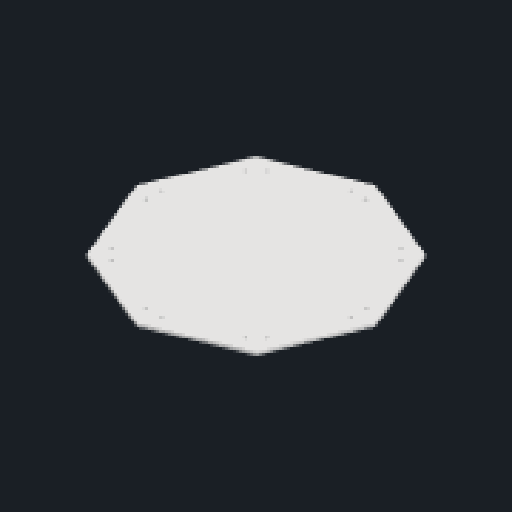
# Autodesk Inventor part: Bund
Saved by Autodesk Inventor 2026.2 (Build 302298000, 298)
## iProperties
Created: 2026-04-22
Part Number: Bund
Material: Generic
Document SubType Name: Modeling
Designer: Mikke
Density: 1 g/cm^3
Appearance: Default
Author: Mikke
Autodesk Inventor part; units mm, degrees
ref_plane "YZ Plane" through (0, 0, 0) normal (1, 0, 0) x (0, 1, 0)
ref_plane "XZ Plane" through (0, 0, 0) normal (0, 1, 0) x (-1, 0, 0)
ref_plane "XY Plane" through (0, 0, 0) normal (0, 0, 1) x (1, 0, 0)
sketch "Sketch1" plane through (0, 0, 0) normal (0, 1, 0) x (-1, 0, 0)
  line L0 (0, 0) -> (0, -104.6)
  line L1 (0, -104.6) -> (-73.9634, -73.9634)
  line L2 (-73.9634, -73.9634) -> (-104.6, 0)
  line L3 (-104.6, 0) -> (-73.9634, 73.9634)
  line L4 (-73.9634, 73.9634) -> (0, 104.6)
  line L5 (0, 104.6) -> (73.9634, 73.9634)
  line L6 (73.9634, 73.9634) -> (104.6, 0)
  line L7 (104.6, 0) -> (73.9634, -73.9634)
  line L8 (73.9634, -73.9634) -> (0, -104.6)
  line L9 (89.2707, -89.2707) -> (126.2478, 0)
  line L10 (126.2478, 0) -> (89.2707, 89.2707)
  line L11 (89.2707, 89.2707) -> (0, 126.2478)
  line L12 (0, 126.2478) -> (-89.2707, 89.2707)
  line L13 (-89.2707, 89.2707) -> (-126.2478, 0)
  line L14 (-126.2478, 0) -> (-89.2707, -89.2707)
  line L15 (-89.2707, -89.2707) -> (0, -126.2478)
  line L16 (0, -126.2478) -> (89.2707, -89.2707)
  line L17 (0, -104.6) -> (7.6537, -123.0776)
  line L18 (0, -104.6) -> (20, -104.6) construction
  line L19 (73.9634, -73.9634) -> (81.617, -92.441)
  line L20 (73.9634, -73.9634) -> (76.2595, -79.5066)
  line L21 (76.2595, -79.5066) -> (70.7162, -81.8027)
  circle A0 centre (70.7162, -81.8027) radius 1.6
  line L22 (0, -104.6) -> (2.2961, -110.1433)
  line L23 (2.2961, -110.1433) -> (7.8394, -107.8472)
  circle A1 centre (7.8394, -107.8472) radius 1.6
  circle A2 centre (107.8472, -7.8394) radius 1.6
  circle A3 centre (81.8027, -70.7162) radius 1.6
  circle A4 centre (81.8027, 70.7162) radius 1.6
  circle A5 centre (107.8472, 7.8394) radius 1.6
  circle A6 centre (7.8394, 107.8472) radius 1.6
  circle A7 centre (70.7162, 81.8027) radius 1.6
  circle A8 centre (-70.7162, 81.8027) radius 1.6
  circle A9 centre (-7.8394, 107.8472) radius 1.6
  circle A10 centre (-107.8472, 7.8394) radius 1.6
  circle A11 centre (-81.8027, 70.7162) radius 1.6
  circle A12 centre (-81.8027, -70.7162) radius 1.6
  circle A13 centre (-107.8472, -7.8394) radius 1.6
  circle A14 centre (-7.8394, -107.8472) radius 1.6
  circle A15 centre (-70.7162, -81.8027) radius 1.6
  dimension "d0" = 104.6
  dimension "d1" = 20
  dimension "d2" = 67.5
  dimension "d3" = 6
  dimension "d4" = 6
  dimension "d5" = 3.2
  dimension "d6" = 6
  dimension "d7" = 3.2
  dimension "d10" = 360
  constraints: 48 end point, 16 centre point, 4 point on line, 3 coincident, 3 perpendicular, 1 equal length, 1 horizontal, 1 vertical, 57 other
  measures "d0" distance of L0.start L0.end
  measures "d1" distance between parallel lines of L7 L9
  measures "d2" angle of L17 L18
  measures "d3" distance of L7.end L20.end
  measures "d4" distance of L20.end L21.end
  measures "d5" diameter of A0
  measures "d6" distance of L22.end L23.end
  measures "d7" diameter of A1
extrude "Extrusion1" add sketch "Sketch1" along normal blind 3
ref_plane "Work Plane1" through (126.2478, 0, 0) normal (0, 0, 1) x (0, 1, 0)
ref_plane "Work Plane2" through (0, 0, -126.2478) normal (1, 0, 0) x (0, 1, 0)
sketch "Sketch3" plane through (0, 0, 0) normal (0, -1, 0) x (1, 0, 0)
  line L0 (-49.9941, -52.4) -> (49.9941, -52.4) construction
  line L1 (49.9941, -52.4) -> (52.4, -49.9941) construction
  line L2 (52.4, -49.9941) -> (52.4, 49.9941) construction
  line L3 (52.4, 49.9941) -> (49.9941, 52.4) construction
  line L4 (49.9941, 52.4) -> (-49.9941, 52.4) construction
  line L5 (-49.9941, 52.4) -> (-52.4, 49.9941) construction
  line L6 (-52.4, 49.9941) -> (-52.4, -49.9941) construction
  line L7 (-52.4, -49.9941) -> (-49.9941, -52.4) construction
  circle A0 centre (-45, -45) radius 1.25 construction
  circle A1 centre (44.8952, -45.0207) radius 1.25 construction
  circle A2 centre (45.9242, 45.9242) radius 1.25 construction
  line L8 (-50.077, 52.6) -> (50.077, 52.6)
  line L9 (50.077, 52.6) -> (52.6, 50.077)
  line L10 (52.6, 50.077) -> (52.6, -50.077)
  line L11 (52.6, -50.077) -> (50.077, -52.6)
  line L12 (50.077, -52.6) -> (-50.077, -52.6)
  line L13 (-50.077, -52.6) -> (-52.6, -50.077)
  line L14 (-52.6, -50.077) -> (-52.6, 50.077)
  line L15 (-52.6, 50.077) -> (-50.077, 52.6)
  point P0 (0, 0)
  dimension "d24" = 0.2
  constraints: 16 end point, 7 other
  measures "d24" distance between parallel lines of L4 L8
extrude "Extrusion3" cut sketch "Sketch3" against normal through all
sketch "Sketch4" plane through (0, 3, 0) normal (0, 1, 0) x (1, 0, 0)
  circle A0 centre (55.9, -37.4) radius 1.75 projected
  circle A1 centre (55.9, 37.4) radius 1.75 projected
  circle A2 centre (-55.9, 37.4) radius 1.75 projected
  circle A3 centre (-55.9, -37.4) radius 1.75 projected
  point P0 (0, 0)
extrude "Extrusion4" cut sketch "Sketch4" against normal blind 10
sketch "Sketch6" plane through (0, 3, 0) normal (0, 1, 0) x (1, 0, 0)
  line L0 (0, 0) -> (-44.6354, -107.7593) construction
  line L1 (-89.2707, -89.2707) -> (0, -126.2478) projected
  line L2 (-33.5487, -120.1907) -> (-19.2967, -85.7831)
  line L3 (-19.2967, -85.7831) -> (-47.013, -74.3026)
  line L4 (-47.013, -74.3026) -> (-61.2651, -108.7102)
  line L5 (-61.2651, -108.7102) -> (-33.5487, -120.1907)
  line L6 (-33.5487, -120.1907) -> (-47.013, -74.3026) construction
  line L7 (-19.2967, -85.7831) -> (-61.2651, -108.7102) construction
  point P0 (-40.2809, -97.2467)
  point P1 (-58.4935, -102.019)
  point P2 (-30.7772, -113.4995)
  dimension "d34" = 30
  dimension "d35" = 30
  constraints: 14 end point, 3 midpoint, 2 parallel, 1 perpendicular, 1 point on line
  measures "d34" distance between parallel lines of L1 L3
  measures "d35" distance between parallel lines of L2 L4
extrude "Extrusion6" cut sketch "Sketch6" against normal blind 10 contours L4 L3 L2 L1
pattern_circular "Circular Pattern1" count 8 over 360 about axis through (0, -10, 0) along (0, 1, 0) of "Extrusion6"
sketch "Sketch7" plane through (0, 3, 0) normal (0, 1, 0) x (1, 0, 0)
  circle A0 centre (-28, -70) radius 1.75
  circle A1 centre (-28, 70) radius 1.75
  line L0 (0, 176.747) -> (0, -176.747) projected
  line L1 (-30.7772, -113.4995) -> (0, -126.2478) projected
  line L2 (0, 126.2478) -> (-30.7772, 113.4995) projected
  line L3 (0, -126.2478) -> (0, 126.2478)
  circle A2 centre (28, -70) radius 1.75
  circle A3 centre (28, 70) radius 1.75
  point P0 (0, 0)
  dimension "d41" = 3.5
  dimension "d42" = 3.5
  dimension "d43" = 70
  dimension "d44" = 70
  dimension "d45" = 28
  dimension "d46" = 28
  constraints: 4 centre point, 2 end point, 2 symmetric about line, 1 vertical, 2 other
  measures "d41" diameter of A0
  measures "d42" diameter of A1
  measures "d43" vertical distance of point (0, 0) A0.centre
  measures "d44" vertical distance of A1.centre point (0, 0)
  measures "d45" horizontal distance of point (0, 0) A0.centre
  measures "d46" distance from line of L0 A1.centre
extrude "Extrusion7" cut sketch "Sketch7" against normal blind 10
body "Solid1"
